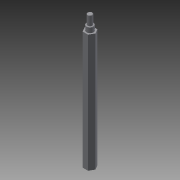
# Autodesk Inventor part: Hex Shaft
Saved by Autodesk Inventor 2013 (Build 170138000, 138)
## iProperties
Created: 2013-01-11
Part Number: Hex Shaft
Material: Generic
Document SubType Name: Modeling
Designer: Naphat
Density: 1 g/cm^3
Author: Naphat
Autodesk Inventor part; units mm, degrees
ref_plane "YZ Plane" through (0, 0, 0) normal (1, 0, 0) x (0, 1, 0)
ref_plane "XZ Plane" through (0, 0, 0) normal (0, 1, 0) x (-1, 0, 0)
ref_plane "XY Plane" through (0, 0, 0) normal (0, 0, 1) x (1, 0, 0)
sketch "Sketch1" plane through (0, 0, 0) normal (0, 1, 0) x (-1, 0, 0)
  line L0 (7.1393, -6.0921) -> (-0.2013, -6.0921)
  line L1 (-0.2013, -6.0921) -> (-3.8716, 0.2651)
  line L2 (-3.8716, 0.2651) -> (-0.2013, 6.6222)
  line L3 (-0.2013, 6.6222) -> (7.1393, 6.6222)
  line L4 (7.1393, -6.0921) -> (10.8096, 0.2651)
  line L5 (10.8096, 0.2651) -> (7.1393, 6.6222)
  point P0 (0, 0)
  dimension "d0" = 7.3406
  dimension "d1" = 7.3406
  dimension "d2" = 7.3406
  dimension "d3" = 7.3406
  dimension "d4" = 120
  dimension "d5" = 120
  dimension "d6" = 120
  dimension "d7" = 7.3406
  dimension "d8" = 120
  dimension "d9" = 7.3406
  constraints: 12 end point, 1 horizontal, 1 parallel
  measures "d0" distance of L0.start L0.end
  measures "d1" distance of L0.end L1.end
  measures "d2" distance of L1.end L2.end
  measures "d3" distance of L2.end L3.end
  measures "d4" angle of L1 L0
  measures "d5" angle of L1 L2
  measures "d6" angle of L3 L2
  measures "d7" distance of L0.start L4.end
  measures "d8" angle of L0 L4
  measures "d9" distance of L4.end L3.end
extrude "Extrusion1" add sketch "Sketch1" along normal blind 254
sketch "Sketch3" plane through (0, 254, 0) normal (0, 1, 0) x (1, 0, 0)
  circle A0 centre (-3.469, -0.2651) radius 4.699
  point P0 (0, 0)
  dimension "d21" = 9.398
  constraints: 1 centre point
  measures "d21" diameter of A0
extrude "Extrusion2" add sketch "Sketch3" along normal blind 7.112
chamfer "Chamfer1" distance 0.5 angle 45 1 edges at (-8.168, 261.112, 0.2651)
sketch "Sketch4" plane through (-3.469, 261.112, 0.2651) normal (0, 1, 0) x (1, 0, 0)
  circle A0 centre (0, 0) radius 4.199 projected
  circle A1 centre (0, 0) radius 3.1877
  point P0 (3.469, 0.2651)
  dimension "d27" = 6.3754
  constraints: 1 centre point, 1 coincident
  measures "d27" diameter of A1
extrude "Extrusion3" add sketch "Sketch4" along normal blind 12.7 contours A1
chamfer "Chamfer2" distance 0.5 angle 45 1 edges at (-6.6567, 273.812, 0.2651)
sketch "Sketch5" plane through (0, 0, 0) normal (0, -1, 0) x (1, 0, 0)
  line L0 (-7.1393, -6.0921) -> (0.2013, -6.0921) projected
  line L1 (0.2013, -6.0921) -> (3.8716, 0.2651) projected
  line L2 (3.8716, 0.2651) -> (0.2013, 6.6222) projected
  line L3 (0.2013, 6.6222) -> (-7.1393, 6.6222) projected
  line L4 (-7.1393, 6.6222) -> (-10.8096, 0.2651) projected
  line L5 (-10.8096, 0.2651) -> (-7.1393, -6.0921) projected
  point P0 (0, 0)
extrude "Extrusion4" cut sketch "Sketch5" against normal blind 101.346
sketch "Sketch6" plane through (0, 101.346, 0) normal (0, -1, 0) x (1, 0, 0)
  line L0 (0.2013, -6.0921) -> (-7.1393, -6.0921) projected
  line L1 (3.8716, 0.2651) -> (0.2013, -6.0921) projected
  line L2 (0.2013, 6.6222) -> (3.8716, 0.2651) projected
  line L3 (-7.1393, 6.6222) -> (0.2013, 6.6222) projected
  line L4 (-10.8096, 0.2651) -> (-7.1393, 6.6222) projected
  line L5 (-7.1393, -6.0921) -> (-10.8096, 0.2651) projected
  point P0 (0, 0)
extrude "Extrusion5" add sketch "Sketch6" along normal blind 7.3406
sketch "Sketch7" plane through (0, 94.0054, 0) normal (0, -1, 0) x (1, 0, 0)
  circle A0 centre (-3.469, 0.2651) radius 2.4892
  point P0 (0, 0)
  dimension "d37" = 4.9784
  constraints: 1 centre point
  measures "d37" diameter of A0
extrude "Extrusion6" cut sketch "Sketch7" against normal blind 15.875
sketch "Sketch8" plane through (-3.469, 109.8804, 0.2651) normal (0, -1, 0) x (1, 0, 0)
  circle A0 centre (0, 0) radius 2.4892 projected
  point P0 (3.469, -0.2651)
fillet "Fillet1" radius 1.3462 1 edges at (-5.9582, 109.8804, 0.2651)
equation "\"d5\" = d4"
equation "\"d8\" = d4"
body "Solid1"
